PLATE_LV_BACK (Autodesk Fusion 360 design; units mm, degrees)
Autodesk Fusion 360 part; units mm, degrees
note: some values were not read from the file. Set by a fixed rule: which sketch regions a step uses.
sketch "Esquisse1" plane through (0, 0, 0) normal (0, 0, 1) x (1, 0, 0)
  line L0 (75, -53) -> (-75, -53)
  line L1 (-75, -53) -> (-75, 53)
  line L2 (-75, 53) -> (75, 53)
  line L3 (75, 53) -> (75, -53)
  line L4 (75, -53) -> (-75, 53) construction
  line L5 (-75, -53) -> (75, 53) construction
  line L6 (78, 50) -> (-78, 50)
  line L7 (-78, 50) -> (-78, -50)
  line L8 (-78, -50) -> (78, -50)
  line L9 (78, -50) -> (78, 50)
  line L10 (78, 50) -> (-78, -50) construction
  line L11 (-78, 50) -> (78, -50) construction
  dimension "d1" = 150
  dimension "d2" = 106
  dimension "d49" = 156
  dimension "d50" = 100
  constraint horizontal L0
  constraint perpendicular L0 L1
  constraint parallel L0 L2
  constraint parallel L1 L3
  constraint coincident L4 origin
  constraint coincident L5 origin
  constraint horizontal L6
  constraint perpendicular L6 L7
  constraint parallel L6 L8
  constraint parallel L7 L9
  constraint coincident L10 origin
  constraint coincident L11 origin
  measures "d1" distance of L1.end L2.end
  measures "d2" distance of L0.end L1.end
  measures "d49" distance of L7.end L8.end
  measures "d50" distance of L6.end L7.end
extrude "Extrusion1" add sketch "Esquisse1" along normal blind 3
sketch "Esquisse4" plane through (0, 0, 3) normal (0, 0, 1) x (-1, 0, 0)
  line L0 (-75, -53) -> (75, -53)
  line L1 (75, -53) -> (75, -50)
  line L2 (75, 53) -> (-75, 53)
  line L3 (-75, -50) -> (-75, -53)
  circle A0 centre (-25, -37.5) radius 2.5
  circle A1 centre (-25, -28.125) radius 2.5
  circle A2 centre (-25, -18.75) radius 2.5
  circle A3 centre (-25, -9.375) radius 2.5
  circle A4 centre (-25, 0) radius 2.5
  circle A5 centre (-12.1742, -35.2385) radius 2.5
  circle A6 centre (-0.8955, -28.7267) radius 2.5
  circle A7 centre (7.476, -18.75) radius 2.5
  circle A8 centre (11.9303, -6.5118) radius 2.5
  circle A9 centre (11.9303, 6.5118) radius 2.5
  circle A10 centre (7.476, 18.75) radius 2.5
  circle A11 centre (-0.8955, 28.7267) radius 2.5
  circle A12 centre (-12.1742, 35.2385) radius 2.5
  circle A13 centre (-25, 37.5) radius 2.5
  circle A14 centre (-37.8258, 35.2385) radius 2.5
  circle A15 centre (-49.1045, 28.7267) radius 2.5
  circle A16 centre (-57.476, 18.75) radius 2.5
  circle A17 centre (-61.9303, 6.5118) radius 2.5
  circle A18 centre (-61.9303, -6.5118) radius 2.5
  circle A19 centre (-57.476, -18.75) radius 2.5
  circle A20 centre (-49.1045, -28.7267) radius 2.5
  circle A21 centre (-37.8258, -35.2385) radius 2.5
  circle A22 centre (-12.797, -25.3397) radius 2.5
  circle A23 centre (-3.011, -17.5357) radius 2.5
  circle A24 centre (2.4198, -6.2584) radius 2.5
  circle A25 centre (2.4198, 6.2584) radius 2.5
  circle A26 centre (-3.011, 17.5357) radius 2.5
  circle A27 centre (-12.797, 25.3397) radius 2.5
  circle A28 centre (-25, 28.125) radius 2.5
  circle A29 centre (-37.203, 25.3397) radius 2.5
  circle A30 centre (-46.989, 17.5357) radius 2.5
  circle A31 centre (-52.4198, 6.2584) radius 2.5
  circle A32 centre (-52.4198, -6.2584) radius 2.5
  circle A33 centre (-46.989, -17.5357) radius 2.5
  circle A34 centre (-37.203, -25.3397) radius 2.5
  circle A35 centre (-13.979, -15.1691) radius 2.5
  circle A36 centre (-7.1677, -5.7941) radius 2.5
  circle A37 centre (-7.1677, 5.7941) radius 2.5
  circle A38 centre (-13.979, 15.1691) radius 2.5
  circle A39 centre (-25, 18.75) radius 2.5
  circle A40 centre (-36.021, 15.1691) radius 2.5
  circle A41 centre (-42.8323, 5.7941) radius 2.5
  circle A42 centre (-42.8323, -5.7941) radius 2.5
  circle A43 centre (-36.021, -15.1691) radius 2.5
  circle A44 centre (-17.6703, -5.8452) radius 2.5
  circle A45 centre (-15.8601, 2.0861) radius 2.5
  circle A46 centre (-20.9323, 8.4466) radius 2.5
  circle A47 centre (-29.0677, 8.4466) radius 2.5
  circle A48 centre (-34.1399, 2.0861) radius 2.5
  circle A49 centre (-32.3297, -5.8452) radius 2.5
  line L4 (-75, 50) -> (-78, 50)
  line L5 (-78, 50) -> (-78, -50)
  line L6 (-78, -50) -> (-75, -50)
  line L7 (75, -50) -> (78, -50)
  line L8 (78, -50) -> (78, 50)
  line L9 (78, 50) -> (75, 50)
  line L10 (75, 50) -> (75, 53)
  line L11 (-75, 53) -> (-75, 50)
  circle A50 centre (-60.75, -35.75) radius 2.2
  circle A51 centre (10.75, 35.75) radius 2.2
  line L12 (-60.75, -35.75) -> (10.75, -35.75)
  line L13 (10.75, 35.75) -> (-60.75, -35.75) construction
  line L14 (-60.75, 35.75) -> (10.75, -35.75) construction
  circle A52 centre (10.75, -35.75) radius 2.2
  line L15 (10.75, 35.75) -> (-60.75, 35.75)
  line L16 (-60.75, 35.75) -> (-60.75, -35.75)
  line L17 (10.75, -35.75) -> (10.75, 35.75)
  circle A53 centre (-60.75, 35.75) radius 2.2
  line L18 (-75, 50) -> (-78, 50)
  point P0 (-25, 0)
  dimension "d32" = 5
  dimension "d37" = 0
  dimension "d38" = 37.5
  dimension "d40" = 360
  dimension "d42" = 360
  dimension "d44" = 360
  dimension "d46" = 360
  dimension "d51" = 71.5
  dimension "d52" = 71.5
  dimension "d53" = 4.4
  dimension "d54" = 4.4
  dimension "d55" = 4.4
  dimension "d56" = 4.4
  constraint horizontal L15
  constraint perpendicular L15 L16
  constraint parallel L12 L15
  constraint parallel L16 L17
  constraint coincident P0 L13
  constraint coincident P0 L14
  constraint coincident A50.centre L12.start
  constraint coincident L14.start L15.end
  constraint coincident A51.centre L13.start
  constraint coincident L12.end L14.end
  constraint coincident P0 A4.centre
  measures "d32" diameter of A0
  measures "d51" distance of A50.centre L14.start
  measures "d52" distance of A50.centre L12.end
  measures "d53" diameter of A50
  measures "d54" diameter of A53
  measures "d55" diameter of A51
  measures "d56" diameter of A52
extrude "Extrusion5" cut sketch "Esquisse4" against normal blind 3 contours A0 L12 | A0 L12 | A5 L12 | A5 L12 | A21 L12 | A21 L12 | L12 A52 L17 | L12 A52 L17 | A50 L12 L16 | A50 L12 L16 | A8 L17 | A8 L17 | A18 L16 | A18 L16 | A9 L17 | A9 L17 | A17 L16 | A17 L16 | A51 L15 L17 | A51 L15 L17 | L15 L16 A53 | L15 L16 A53 | A12 L15 | A12 L15 | A14 L15 | A14 L15 | A13 L15 | A13 L15 | A1 | A2 | A3 | A4 | A6 | A7 | A10 | A11 | A15 | A16 | A19 | A20 | A22 | A23 | A24 | A25 | A26 | A27 | A28 | A29 | A30 | A31 | A32 | A33 | A34 | A35 | A36 | A37 | A38 | A39 | A40 | A41 | A42 | A43 | A44 | A45 | A46 | A47 | A48 | A49
